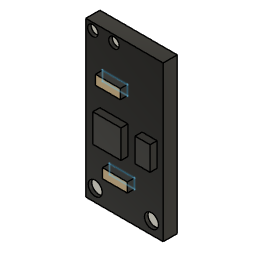
DC-DC+down (Autodesk Fusion 360 design; units mm, degrees)
Autodesk Fusion 360 part; units mm, degrees
sketch "Boceto1" plane through (0, 0, 0) normal (0, 1, 0) x (1, 0, 0)
  line L0 (0, 0) -> (11, 0)
  line L1 (11, 0) -> (11, -22)
  line L2 (11, -22) -> (0, -22)
  line L3 (0, -22) -> (0, 0)
  dimension "d1" = 11
  dimension "d2" = 22
  constraint horizontal L0
  constraint vertical L1
  constraint horizontal L2
  constraint vertical L3
  constraint coincident L0.start L3.end
  measures "d1" distance of L0.start L0.end
  measures "d2" distance of L0.start L2.end
extrude "Extruir1" add sketch "Boceto1" along normal blind 2
sketch "Boceto2" plane through (0, 0, 0) normal (0, -1, 0) x (1, 0, 0)
  line L0 (11, 22) -> (0, 22)
  line L1 (0, 22) -> (0, 0)
  line L2 (0, 0) -> (11, 0)
  line L3 (11, 0) -> (11, 22)
  line L4 (8, 12) -> (10.1306, 12)
  line L5 (10.1306, 12) -> (10.1306, 8.6002)
  line L6 (10.1306, 8.6002) -> (8, 8.6002)
  line L7 (8, 8.6002) -> (8, 12)
  line L8 (2, 12) -> (6, 12)
  line L9 (6, 12) -> (6, 8)
  line L10 (6, 8) -> (2, 8)
  line L11 (2, 8) -> (2, 12)
  constraint horizontal L4
  constraint vertical L5
  constraint horizontal L6
  constraint vertical L7
  constraint horizontal L8
  constraint vertical L9
  constraint horizontal L10
  constraint vertical L11
extrude "Extruir2" add sketch "Boceto2" along normal blind 1 contours L4 L5 L6 L7 | L8 L9 L10 L11
sketch "Boceto3" plane through (0, 0, 0) normal (0, 1, 0) x (1, 0, 0)
  circle A0 centre (1.3364, -1.7459) radius 0.9984
  circle A1 centre (9.3364, -1.7459) radius 0.9984
  circle A2 centre (1, -21) radius 0.7455
  circle A3 centre (4, -21) radius 0.7455
extrude "Extruir3" cut sketch "Boceto3" along normal blind 0.5
sketch "Boceto4" plane through (0, 0, 0) normal (0, 1, 0) x (1, 0, 0)
  line L0 (3.3729, -5.8021) -> (6.9064, -5.8021)
  line L1 (6.9064, -5.8021) -> (6.9064, -4.4369)
  line L2 (6.9064, -4.4369) -> (3.3729, -4.4369)
  line L3 (3.3729, -4.4369) -> (3.3729, -5.8021)
  line L4 (2.3729, -16.8021) -> (5.9064, -16.8021)
  line L5 (5.9064, -15.4369) -> (2.3729, -15.4369)
  line L6 (2.3729, -15.4369) -> (2.3729, -16.8021)
  line L7 (5.9064, -16.8021) -> (5.9064, -15.4369)
  constraint horizontal L0
  constraint vertical L1
  constraint horizontal L2
  constraint vertical L3
  constraint horizontal L4
  constraint vertical L7
  constraint horizontal L5
  constraint vertical L6
extrude "Extruir5" add sketch "Boceto4" against normal blind 1
